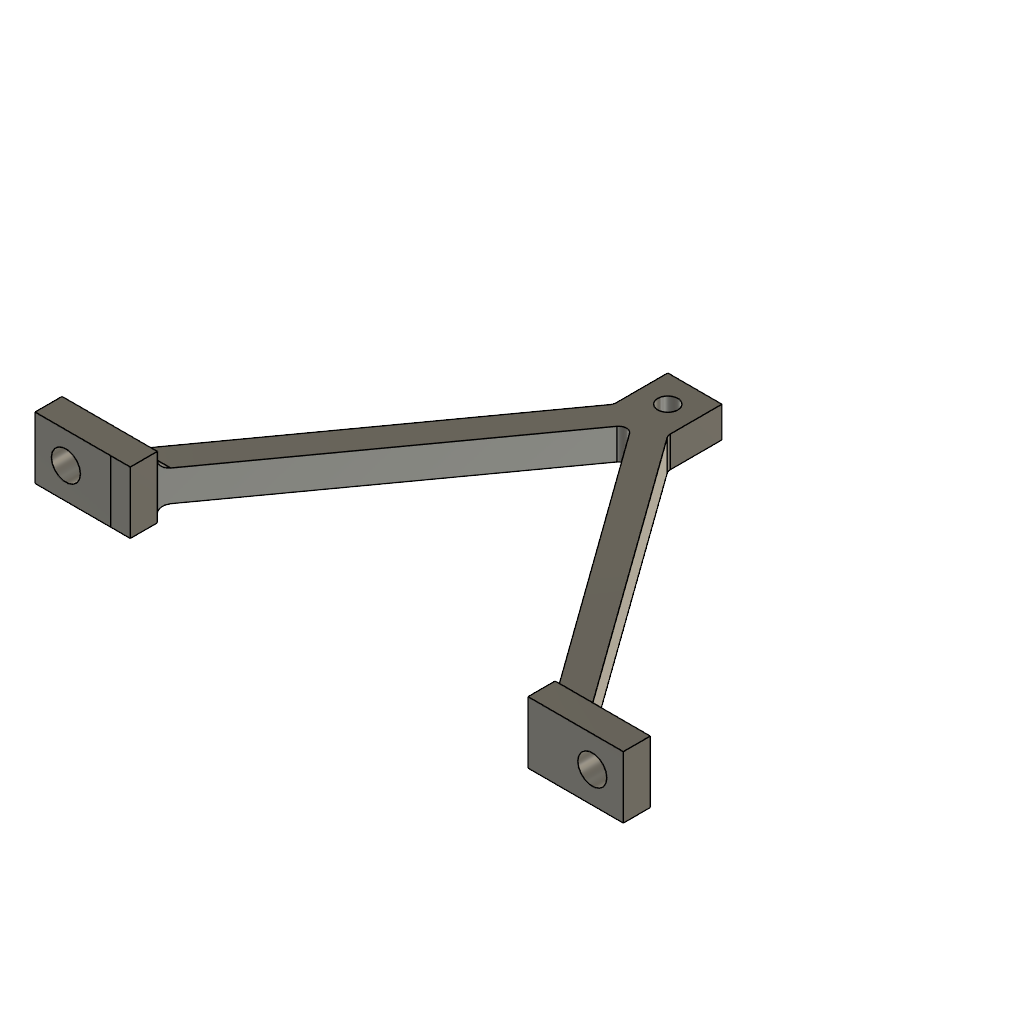
Gantry Support (Autodesk Fusion 360 design; units mm, degrees)
part number: 2026-09-14-21-03-58-136
Autodesk Fusion 360 part; units mm, degrees
sketch "Sketch1" plane through (0, 0, 0) normal (0, 0, 1) x (1, 0, 0)
  line L0 (0, 0) -> (8, 0)
  line L1 (8, 0) -> (38, 0) construction
  line L2 (38, 0) -> (38, 40.25) construction
  circle A0 centre (38, 40.25) radius 1.3
  line L3 (41.5, 36.75) -> (34.5, 36.75)
  line L4 (34.5, 36.75) -> (34.5, 43.75)
  line L5 (34.5, 43.75) -> (41.5, 43.75)
  line L6 (41.5, 43.75) -> (41.5, 36.75)
  line L7 (41.5, 36.75) -> (34.5, 43.75) construction
  line L8 (34.5, 36.75) -> (41.5, 43.75) construction
  line L9 (8, 0) -> (34.5, 36.75)
  line L10 (38, 0) -> (68, 0) construction
  line L11 (68, 0) -> (76, 0)
  line L12 (68, 0) -> (41.5, 36.75)
  line L13 (76, 0) -> (76, -3.5)
  line L14 (76, -3.5) -> (68, -3.5)
  line L15 (0, 0) -> (0, -3.5)
  line L16 (0, -3.5) -> (8, -3.5)
  line L17 (11.2549, 4.5139) -> (14.0938, 2.4668) construction
  line L18 (8, -3.5) -> (9.7912, -3.5)
  line L19 (14.0938, 2.4668) -> (38, 35.6197)
  line L20 (65.1473, 3.9562) -> (62.3083, 1.9091) construction
  line L21 (62.3083, 1.9091) -> (38, 35.6197)
  line L22 (68, -3.5) -> (66.2088, -3.5)
  line L23 (8, 0) -> (12.315, 0)
  line L24 (68, 0) -> (63.685, 0)
  line L25 (14.0938, 2.4668) -> (12.315, 0)
  line L26 (12.315, 0) -> (12.315, -3.5)
  line L27 (12.315, -3.5) -> (9.7912, -3.5)
  line L28 (62.3083, 1.9091) -> (63.685, 0)
  line L29 (63.685, 0) -> (63.685, -3.5)
  line L30 (66.2088, -3.5) -> (63.685, -3.5)
  point P0 (38, 40.25)
  dimension "d1" = 8
  dimension "d2" = 30
  dimension "d3" = 40.25
  dimension "d4" = 2.6
  dimension "d5" = 7
  dimension "d6" = 7
  dimension "d7" = 30
  dimension "d8" = 8
  dimension "d9" = 3.5
  dimension "d10" = 3.5
  constraint coincident L0.start L15.start
  constraint horizontal L0
  constraint horizontal L1
  constraint perpendicular L1 L2
  constraint coincident P0 L2.end
  constraint horizontal L3
  constraint perpendicular L3 L4
  constraint parallel L3 L5
  constraint parallel L4 L6
  constraint coincident L7 P0
  constraint coincident L8 P0
  constraint perpendicular L2 L10
  constraint perpendicular L2 L11
  constraint perpendicular L11 L13
  constraint perpendicular L13 L14
  constraint perpendicular L0 L15
  constraint perpendicular L15 L16
  constraint coincident L9 L17.start
  constraint perpendicular L9 L17
  constraint parallel L16 L18
  constraint coincident L2 L19.end
  constraint perpendicular L17 L19
  constraint coincident L12 L20.start
  constraint perpendicular L12 L20
  constraint perpendicular L20 L21
  constraint parallel L14 L22
  constraint coincident L1 L23.end
  constraint coincident L10 L24.end
  constraint perpendicular L17 L25
  constraint perpendicular L23 L26
  constraint perpendicular L20 L28
  constraint perpendicular L29 L30
  measures "d1" distance of L0.start L0.end
  measures "d2" distance of L0.end L1.end
  measures "d3" distance of L1.end P0
  measures "d4" diameter of A0
  measures "d5" distance of L4.end L5.end
  measures "d6" distance of L3.end L4.end
  measures "d7" distance of L1.end L10.end
  measures "d8" distance of L10.end L11.end
  measures "d9" distance of L11.end L13.end
  measures "d10" distance of L0.start L15.end
extrude "Extrude1" add sketch "Sketch1" along normal blind 4 contours L3 L9 L12 L19 L21 L23 L24 L25 L28 | L3 L4 L5 L6 makes body 1
extrude "Extrude2" add sketch "Sketch1" along normal blind 6 separate body contours L0 L15 L16 L18 L23 L26 L27 | L11 L13 L14 L22 L24 L29 L30 makes body 2 at (67.79, 0, 2) makes body 3 at (4.105, 0, 2)
extrude "Extrude3" add sketch "Sketch1" against normal blind 2 contours L0 L15 L16 L18 L23 L26 L27 | L11 L13 L14 L22 L24 L29 L30 bodies 1 2 3
sketch "Sketch2" plane through (0, 0, 0) normal (0, 1, 0) x (-1, 0, 0)
  line L0 (-12.315, 4) -> (-8, 4)
  line L1 (-8, 4) -> (-8, 0)
  line L2 (-8, 0) -> (-12.315, 0)
  line L3 (-12.315, -2) -> (0, -2)
  line L4 (0, -2) -> (0, 6)
  line L5 (0, 6) -> (-12.315, 6)
  line L6 (-8.0111, 1.6089) -> (0, 2) construction
  line L7 (-4, 6) -> (-4, -2) construction
  circle A0 centre (-4, 2) radius 1.875
  line L8 (-12.315, 0) -> (-12.315, -2)
  line L9 (-12.315, 6) -> (-12.315, 4)
  dimension "d19" = 4
  dimension "d20" = 3.75
  constraint midpoint L4 L6.end
  constraint coincident L5 L7.start
  constraint coincident L3 L7.end
  constraint perpendicular L3 L7
  constraint midpoint L7 A0.centre
  measures "d19" distance of L4 L7
  measures "d20" diameter of A0
extrude "Extrude4" cut sketch "Sketch2" against normal blind 3.5 contours A0 bodies 1
sketch "Sketch3" plane through (0, 0, 0) normal (0, 1, 0) x (-1, 0, 0)
  line L0 (-68, 4) -> (-63.685, 4)
  line L1 (-63.685, 4) -> (-63.685, 6)
  line L2 (-63.685, 6) -> (-76, 6)
  line L3 (-76, 6) -> (-76, -2)
  line L4 (-76, -2) -> (-63.685, -2)
  line L5 (-63.685, -2) -> (-63.685, 0)
  line L6 (-63.685, 0) -> (-68, 0)
  line L7 (-68, 0) -> (-68, 4)
  line L8 (-76, 2) -> (-68, 2) construction
  line L9 (-72, 6) -> (-72, -2) construction
  circle A0 centre (-72, 2) radius 1.875
  dimension "d23" = 4
  dimension "d24" = 3.75
  constraint midpoint L3 L8.start
  constraint midpoint L7 L8.end
  constraint coincident L2 L9.start
  constraint coincident L4 L9.end
  constraint perpendicular L4 L9
  constraint midpoint L8 A0.centre
  measures "d23" distance of L3 L9
  measures "d24" diameter of A0
extrude "Extrude5" cut sketch "Sketch3" against normal blind 3.5 contours A0 bodies 1
fillet "Fillet1" radius 1 2 edges at (41.5, 36.75, 2) (34.5, 36.75, 2) on bodies 1
fillet "Fillet2" radius 1 3 edges at (68, 0, 2) (65.8425, 0, 0) (65.8425, 0, 4) on bodies 1
fillet "Fillet3" radius 1 3 edges at (8, 0, 2) (10.1575, 0, 4) (10.1575, 0, 0) on bodies 1
fillet "Fillet4" radius 1 1 edges at (38, 35.6197, 2) on bodies 1
